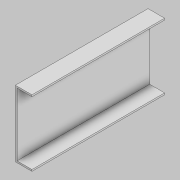
# Autodesk Inventor part: VerseFrameCChannel 4in
Saved by Autodesk Inventor 2021 (Build 250183000, 183)
## iProperties
Created: 2021-02-26
Part Number: VerseFrameCChannel 4in
Material: Generic
Document SubType Name: Modeling
Designer: Merkileg
Density: 1 g/cm^3
Appearance: Default
Author: Merkileg
Autodesk Inventor part; units mm, degrees
ref_plane "YZ Plane" through (0, 0, 0) normal (1, 0, 0) x (0, 1, 0)
ref_plane "XZ Plane" through (0, 0, 0) normal (0, 1, 0) x (-1, 0, 0)
ref_plane "XY Plane" through (0, 0, 0) normal (0, 0, 1) x (1, 0, 0)
sketch "Sketch1" plane through (0, 0, 0) normal (0, 0, 1) x (1, 0, 0)
  line L0 (0, 0) -> (12.7, 0)
  line L1 (12.7, 50.8) -> (0, 50.8)
  line L2 (0, 50.8) -> (0, 0)
  line L3 (12.7, 1.27) -> (1.27, 1.27)
  line L4 (1.27, 1.27) -> (1.27, 49.53)
  line L5 (1.27, 49.53) -> (12.7, 49.53)
  line L6 (12.7, 0) -> (12.7, 1.27)
  line L7 (12.7, 49.53) -> (12.7, 50.8)
  dimension "d0" = 12.7
  dimension "d1" = 50.8
  dimension "d2" = 11.43
  dimension "d3" = 48.26
  constraints: 16 end point, 6 perpendicular, 3 parallel, 1 horizontal
  measures "d0" distance of L1.end L1.start
  measures "d1" distance of L1.start L0.end
  measures "d2" distance of L3.start L3.end
  measures "d3" distance of L3.end L4.end
extrude "Extrusion1" add sketch "Sketch1" along normal blind 101.6
equation "\"d4\" = u1"
equation "\"u1\" = 101.6"
body "Solid1"
